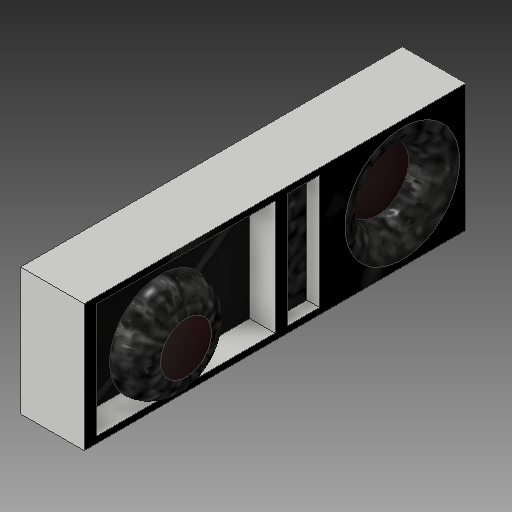
# Autodesk Inventor part: 红外测距
Saved by Autodesk Inventor 2017 (Build 210142000, 142)
## iProperties
Part Number: 红外测距
Material: 常规
Document SubType Name: Modeling
Designer: PANDA
Density: 1 g/cm^3
Appearance: 默认
Mass: 1.2517 g
Surface Area: 12.6215 cm^2
Volume: 1.2517 cm^3
Author: PANDA
Autodesk Inventor part; units mm, degrees
ref_plane "YZ Plane" through (0, 0, 0) normal (1, 0, 0) x (0, 1, 0)
ref_plane "XZ Plane" through (0, 0, 0) normal (0, 1, 0) x (-1, 0, 0)
ref_plane "XY Plane" through (0, 0, 0) normal (0, 0, 1) x (1, 0, 0)
sketch "草图1" plane through (0, 0, 0) normal (1, 0, 0) x (0, 1, 0)
  line L0 (5, 15) -> (-5, 15)
  line L1 (-5, 15) -> (-5, -15)
  line L2 (-5, -15) -> (5, -15)
  line L3 (5, -15) -> (5, 15)
  point P0 (0, 0)
  dimension "d0" = 10
  dimension "d1" = 30
  constraints: 8 end point, 2 parallel, 1 horizontal, 1 perpendicular
  measures "d0" distance of L2.end L1.end
  measures "d1" distance of L1.end L0.end
extrude "拉伸1" add sketch "草图1" along normal blind 5
sketch "草图2" plane through (5, 0, 0) normal (1, 0, 0) x (0, 0, -1)
  line L0 (1, 4.5) -> (3.5, 4.5)
  line L1 (3.5, 4.5) -> (3.5, -4.5)
  line L2 (3.5, -4.5) -> (1, -4.5)
  line L3 (1, -4.5) -> (1, 4.5)
  point P0 (0, 0)
  dimension "d4" = 2.5
  dimension "d5" = 9
  constraints: 8 end point, 2 parallel, 1 horizontal, 1 perpendicular
  measures "d4" distance of L1.end L2.end
  measures "d5" distance of L0.end L1.end
extrude "拉伸2" cut sketch "草图2" against normal blind 1
sketch "草图3" plane through (5, 0, 0) normal (1, 0, 0) x (0, 0, -1)
  circle A0 centre (10, 0) radius 2.5
  point P0 (0, 0)
  dimension "d8" = 5
  constraints: 1 centre point
  measures "d8" diameter of A0
extrude "拉伸3" cut sketch "草图3" against normal blind 2
fillet "圆角1" radius 2 1 edges at (5, 0, -7.5)
sketch "草图4" plane through (5, 0, 0) normal (1, 0, 0) x (0, 0, -1)
  line L0 (-14, 4.5) -> (0, 4.5)
  line L1 (0, 4.5) -> (0, -4.5)
  line L2 (0, -4.5) -> (-14, -4.5)
  line L3 (-14, -4.5) -> (-14, 4.5)
  circle A0 centre (-8.9997, 0) radius 4
  line L4 (-14, 4.5) -> (0, 4.5)
  line L5 (0, 4.5) -> (0, -4.5)
  line L6 (0, -4.5) -> (-14, -4.5)
  line L7 (-14, -4.5) -> (-14, 4.5)
  point P0 (0, 0)
  dimension "d12" = 9
  dimension "d13" = 8
  constraints: 16 end point, 4 parallel, 2 horizontal, 2 perpendicular, 1 centre point
  measures "d12" distance of L0.end L1.end
  measures "d13" diameter of A0
sketch "草图5" plane through (5, 0, 0) normal (1, 0, 0) x (0, 0, -1)
  line L0 (-14, 4.5) -> (0, 4.5)
  line L1 (0, 4.5) -> (0, -4.5)
  line L2 (0, -4.5) -> (-14, -4.5)
  line L3 (-14, -4.5) -> (-14, 4.5)
  point P0 (0, 0)
  dimension "d14" = 14
  dimension "d15" = 9
  constraints: 8 end point, 2 parallel, 1 horizontal, 1 perpendicular
  measures "d14" distance of L1.end L2.end
  measures "d15" distance of L0.end L1.end
extrude "拉伸4" cut sketch "草图5" against normal blind 2
extrude "拉伸5" add sketch "草图4" along normal blind 2 contours A0
fillet "圆角2" radius 2 1 edges at (7, 0, 12.9997)
